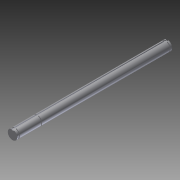
# Autodesk Inventor part: vertical drive shaft 2
Saved by Autodesk Inventor 2012 (Build 160160000, 160)
## iProperties
Created: 2013-01-02
Part Number: vertical drive shaft 2
Material: Default
Document SubType Name: Modeling
Designer: Bryce
Density: 1 g/cm^3
Author: Bryce
Autodesk Inventor part; units mm, degrees
ref_plane "YZ Plane" through (0, 0, 0) normal (1, 0, 0) x (0, 1, 0)
ref_plane "XZ Plane" through (0, 0, 0) normal (0, 1, 0) x (-1, 0, 0)
ref_plane "XY Plane" through (0, 0, 0) normal (0, 0, 1) x (1, 0, 0)
sketch "Sketch1" plane through (0, 0, 0) normal (0, 0, 1) x (1, 0, 0)
  arc A0 (-1, 4.6563) -> (1, 4.6563) centre (0, 0) ccw
  line L0 (-1, 3.7625) -> (1, 3.7625)
  line L1 (1, 3.7625) -> (1, 4.6563)
  line L2 (1, 5.7625) -> (-1, 5.7625) construction
  line L3 (-1, 5.7625) -> (-1, 4.6563) construction
  arc A1 (1, 4.6563) -> (-1, 4.6563) centre (0, 0) ccw construction
  line L4 (-1, 4.6563) -> (-1, 3.7625)
  line L5 (1, 4.6563) -> (1, 5.7625) construction
  dimension "d0" = 9.525
  dimension "d3" = 2
  dimension "d4" = 2
  dimension "d5" = 1
  dimension "d6" = 3.7625
  constraints: 12 end point, 5 parallel, 4 point on circle, 2 centre point, 2 perpendicular, 1 coincident, 1 horizontal
  measures "d0" diameter of A0
  measures "d3" distance of L2.start L2.end
  measures "d4" distance of L0.end L2.start
  measures "d5" distance from line of point (0, 0) L1
  measures "d6" distance from line of point (0, 0) L0
extrude "Extrusion1" add sketch "Sketch1" along normal blind 155.575
ref_plane "Work Plane1" through (0, 0, 1.5875) normal (0, 0, -1) x (-1, 0, 0)
sketch "Sketch2" plane through (0, 0, 1.5875) normal (0, 0, -1) x (-1, 0, 0)
  line L0 (-1, 3.7625) -> (-1, 4.6563) projected
  line L1 (1, 3.7625) -> (-1, 3.7625) projected
  line L2 (1, 4.6563) -> (1, 3.7625) projected
  arc A0 (-1, 4.6563) -> (1, 4.6563) centre (0, 0) ccw projected
  arc A1 (-1, 3.8735) -> (1, 3.8735) centre (0, 0) ccw
  arc A2 (1, 3.8735) -> (-1, 3.8735) centre (0, 0) ccw construction
  dimension "d9" = 0.762
  constraints: 4 point on circle, 2 centre point, 2 point on line, 1 coincident
  measures "d9" radial gap between concentric circles of A1 A0
extrude "Extrusion2" cut sketch "Sketch2" against normal blind 0.762 contours A1 L2 A0 L0
ref_plane "Work Plane2" through (0, 0, 130.683) normal (0, 0, -1) x (-1, 0, 0)
sketch "Sketch3" plane through (0, 0, 130.683) normal (0, 0, -1) x (-1, 0, 0)
  arc A0 (-1, 3.8735) -> (1, 3.8735) centre (0, 0) ccw projected
  line L0 (-1, 3.7625) -> (-1, 4.6563) projected
  arc A1 (-1, 4.6563) -> (1, 4.6563) centre (0, 0) ccw projected
  line L1 (1, 4.6563) -> (1, 3.7625) projected
  line L2 (1, 3.7625) -> (-1, 3.7625) projected
extrude "Extrusion3" cut sketch "Sketch3" against normal blind 0.762 contours A0 L1 A1 L0
ref_plane "Work Plane3" through (0, 0, 153.9875) normal (0, 0, 1) x (1, 0, 0)
sketch "Sketch4" plane through (0, 0, 153.9875) normal (0, 0, 1) x (1, 0, 0)
  arc A0 (-1, 3.8735) -> (1, 3.8735) centre (0, 0) ccw projected
  line L0 (-1, 3.7625) -> (1, 3.7625) projected
  line L1 (-1, 4.6563) -> (-1, 3.7625) projected
  line L2 (1, 3.7625) -> (1, 4.6563) projected
  arc A1 (-1, 4.6563) -> (1, 4.6563) centre (0, 0) ccw projected
extrude "Extrusion4" cut sketch "Sketch4" against normal blind 1.016 contours A0 L2 A1 L1
equation "\"d4\" = d3"
equation "\"d5\" = 0.5 * d3"
equation "\"d6\" = 0.5 * d0 - 0.5 * d4"
body "Solid1"
